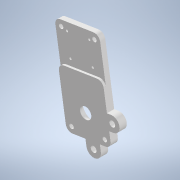
# Autodesk Inventor part: Пластина 1
Saved by Autodesk Inventor 2020 (Build 240168000, 168)
## iProperties
Created: 2020-12-07
Part Number: Пластина 1
Material: Типовые
Document SubType Name: Modeling
Designer: User
Density: 1 g/cm^3
Appearance: По умолчанию
Author: User
Autodesk Inventor part; units mm, degrees
ref_plane "YZ Plane" through (0, 0, 0) normal (1, 0, 0) x (0, 1, 0)
ref_plane "XZ Plane" through (0, 0, 0) normal (0, 1, 0) x (-1, 0, 0)
ref_plane "XY Plane" through (0, 0, 0) normal (0, 0, 1) x (1, 0, 0)
sketch "Эскиз1" plane through (0, 0, 0) normal (0, 0, 1) x (1, 0, 0)
  circle A0 centre (0, 0) radius 14 projected
  circle A1 centre (-4.693, 29.6307) radius 12 projected
  line L0 (15.6838, 99.782) -> (35.4101, -24.7655)
  line L1 (35.4101, -24.7655) -> (-26.0241, -34.4958)
  line L2 (-26.0241, -34.4958) -> (-45.7505, 90.0517)
  line L3 (-45.7505, 90.0517) -> (15.6838, 99.782)
  line L4 (7.1366, 89.8223) -> (12.6431, 55.0556) construction
  line L5 (-31.6345, 87.2252) -> (3.1321, 92.7317) construction
  line L6 (-29.0374, 48.4541) -> (-34.5439, 83.2207) construction
  point P0 (0, 0)
  dimension "d0" = 10
  dimension "d1" = 10
  dimension "d2" = 5
  dimension "d3" = 30
  constraints: 8 end point, 4 parallel, 1 perpendicular
  measures "d0" distance between parallel lines of L0 L4
  measures "d1" distance between parallel lines of L2 L6
  measures "d2" distance between parallel lines of L3 L5
  measures "d3" distance from line of L1 A0.centre
ref_plane "РабПлоскость1" through (-35.2416, 44.847, 7) normal (0, 0, -1) x (-0.1564345, 0.9876883, 0)
extrude "Выдавливание1" add sketch "Эскиз1" along normal up to surface (7 mm away)
sketch "Эскиз2" plane through (35.4101, -24.7655, 7) normal (0, 0, 1) x (0.9876883, 0.1564345, 0)
  circle A0 centre (-31.1, 60) radius 12 projected
  point P0 (-31.1, 30)
ref_plane "РабПлоскость2" through (-17.9323, 16.3914, 6) normal (0, 0, 1) x (0.9876885, 0.1564338, 0)
extrude "Выдавливание2" add sketch "Эскиз2" against normal up to surface (1 mm away)
sketch "Эскиз3" plane through (35.4101, -24.7655, 7) normal (0, 0, 1) x (0.9876883, 0.1564345, 0)
  line L0 (-62.2, 126.1) -> (-62.2, 0) projected
  line L1 (0, 0) -> (0, 126.1) projected
  line L2 (-62.2, 0) -> (0, 0)
  line L3 (0, 0) -> (0, 75.9)
  line L4 (0, 75.9) -> (-62.2, 75.9)
  line L5 (-62.2, 75.9) -> (-62.2, 0)
  line L6 (-13.5, 78.9) -> (-48.7, 78.9) construction
  circle A0 centre (-31.1, 30) radius 7.5 projected
  point P0 (-31.1, 30)
  point P1 (0, 0)
  point P2 (-62.2, 75.9)
  dimension "d8" = 3
  constraints: 8 end point, 2 parallel, 1 horizontal, 1 perpendicular, 1 point on line
  measures "d8" distance between parallel lines of L6 L4
ref_plane "РабПлоскость3" through (-9.421, -9.421, 10) normal (0, 0, 1) x (1, 0, 0)
extrude "Выдавливание3" add sketch "Эскиз3" along normal up to surface (3 mm away)
fillet "Сопряжение1" radius 0.5 1 edges at (-7.4077, -1.1733, 10)
fillet "Сопряжение2" radius 8 6 edges at (-45.7505, 90.0517, 3.5) (-26.0241, -34.4958, 5) (35.4101, -24.7655, 5) (15.6838, 99.782, 3.5) (23.5368, 50.2, 8.5) (-37.8974, 40.4698, 8.5)
sketch "Эскиз4" plane through (0, 0, 0) normal (0, 0, -1) x (-1, 0, 0)
  arc A0 (-7.7822, 98.5305) -> (-16.9352, 91.8805) centre (-9.0337, 90.629) ccw construction
  arc A1 (44.499, 82.1502) -> (37.849, 91.3032) centre (36.5975, 83.4017) ccw construction
  arc A2 (18.1226, -33.2443) -> (27.2755, -26.5943) centre (19.374, -25.3428) ccw construction
  arc A3 (-34.1587, -16.864) -> (-27.5086, -26.017) centre (-26.2572, -18.1155) ccw construction
  point P0 (0, 0)
hole "Отверстие1" at (26.2572, -18.1155, 0) at (-19.374, -25.3428, 0) at (-36.5975, 83.4017, 0) at (9.0337, 90.629, 0) direction (0, 0, 1) diameter 6 end through all clearance for "с потайной головкой ГОСТ 12876-67" size "M6" standard "ГОСТ"
sketch "Эскиз5" plane through (0, 0, 0) normal (0, 0, -1) x (-1, 0, 0)
  circle A0 centre (23.8348, 51.4043) radius 1.5 construction
  circle A1 centre (-6.7835, 56.2537) radius 1.5 construction
  circle A2 centre (-1.934, 86.8721) radius 1.5 construction
  circle A3 centre (28.6843, 82.0226) radius 1.5 construction
  point P0 (0, 0)
hole "Отверстие2" at (-23.8348, 51.4043, 0) at (-28.6843, 82.0226, 0) at (1.934, 86.8721, 0) at (6.7835, 56.2537, 0) direction (0, 0, 1) diameter 3 end through all countersink diameter 6.6 countersink angle 90 clearance for "с потайной головкой ГОСТ 12876-67" size "M3" standard "ГОСТ"
sketch "Эскиз6" plane through (0, 0, 0) normal (0, 0, -1) x (-1, 0, 0)
  line L0 (-31.1854, 39.6237) -> (-41.9794, -28.5268) construction
  line L1 (-38.6544, -33.1033) -> (16.6561, -41.8636) construction
  circle A0 centre (-36.5824, 5.5484) radius 4
  circle A1 centre (-10.9991, -37.4835) radius 4
  arc A2 (-35.0181, 15.4253) -> (-38.1468, -4.3285) centre (-36.5824, 5.5484) ccw
  line L2 (-38.1468, -4.3285) -> (-32.3194, -5.2514)
  line L3 (-35.0181, 15.4253) -> (-29.1907, 14.5023)
  arc A3 (-20.876, -35.9191) -> (-1.1222, -39.0478) centre (-10.9991, -37.4835) ccw
  line L4 (-20.876, -35.9191) -> (-19.5084, -27.2841)
  line L5 (-1.1222, -39.0478) -> (0.2454, -30.4128)
  line L6 (-27.5086, -26.017) -> (18.1226, -33.2443) projected
  line L7 (-34.1587, -16.864) -> (-16.9352, 91.8805) projected
  point P0 (0, 0)
  point P1 (-38.1468, -4.3285)
  dimension "d27" = 8
  dimension "d28" = 8
  dimension "d29" = 10
  dimension "d30" = 10
  dimension "d31" = 10
  constraints: 8 end point, 4 centre point, 4 perpendicular, 4 point on circle, 4 point on line, 2 coincident, 2 midpoint, 1 parallel
  measures "d27" diameter of A0
  measures "d28" diameter of A1
  measures "d29" radius of A2
  measures "d30" distance from line of A0.centre L2
  measures "d31" radius of A3
extrude "Выдавливание4" add sketch "Эскиз6" against normal up to surface (10 mm away)
equation "\"d28\" = d27"
equation "\"d30\" = d29"
equation "\"d31\" = d29"
